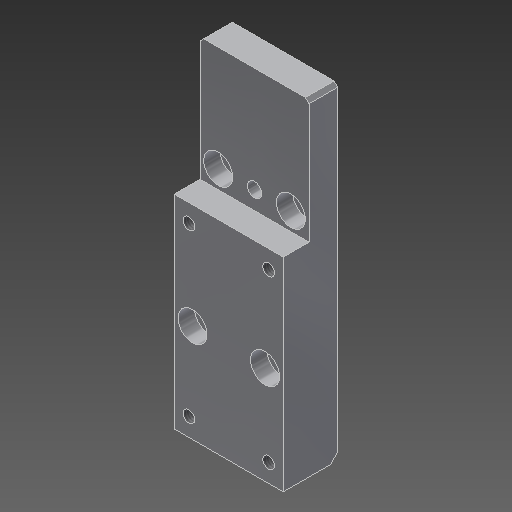
# Autodesk Inventor part: 04
Saved by Autodesk Inventor 2021.1 (Build 251245010, 245A)
## iProperties
Created: 2008-11-14
Part Number: 04
Document SubType Name: Modeling
Density: 2.71 g/cm^3
Material: A5052
Mass: 48.5632 g
Surface Area: 53.44 cm^2
Volume: 17.92 cm^3
Appearance: アルミニウム - フラット
個数: 1
尺度: 1:1
Title: プレート
Autodesk Inventor part; units mm, degrees
ref_plane "YZ Plane" through (0, 0, 0) normal (1, 0, 0) x (0, 1, 0)
ref_plane "XZ Plane" through (0, 0, 0) normal (0, 1, 0) x (-1, 0, 0)
ref_plane "XY Plane" through (0, 0, 0) normal (0, 0, 1) x (1, 0, 0)
sketch "スケッチ1" plane through (0, 0, 0) normal (0, 0, 1) x (1, 0, 0)
  line L0 (-15, -45) -> (15, -45)
  line L1 (15, -45) -> (15, 45)
  line L2 (15, 45) -> (-15, 45)
  line L3 (-15, 45) -> (-15, -45)
  point P0 (0, 0)
  point P1 (0, -45)
  point P2 (-15, 0)
  dimension "d0" = 30
  dimension "d1" = 90
  constraints: 8 end point, 2 midpoint, 2 parallel, 1 horizontal, 1 horizontal alignment, 1 perpendicular, 1 vertical alignment
  measures "d0" distance of L0.start L0.end
  measures "d1" distance of L2.end L0.start
extrude "押し出し1" add sketch "スケッチ1" along normal blind 15
sketch "スケッチ6" plane through (0, 0, 15) normal (0, 0, 1) x (1, 0, 0)
  line L0 (15, -45) -> (-15, -45) projected
  point P0 (0, 0)
  point P1 (-11, -40)
  dimension "d33" = 11
  dimension "d52" = 5
  measures "d33" horizontal distance of point (-11, -40) point (0, 0)
  measures "d52" distance from line of point (-11, -40) L0
hole "穴3" at (-11, -40, 15) direction (0, 0, -1) diameter 3.242 end through all thread size "M4x0.7" class "6H" standard "ANSI Metric M Profile"
pattern_linear "矩形状パターン2" count 2 spacing 22 along (1, 0, 0) count 2 spacing 46 along (0, 1, 0) of "穴3"
sketch "スケッチ9" plane through (0, 0, 15) normal (0, 0, 1) x (1, 0, 0)
  line L0 (15, -45) -> (-15, -45) projected
  point P0 (0, 0)
  point P1 (-10, -18)
  point P2 (10, -18)
  dimension "d53" = 27
  dimension "d54" = 10
  dimension "d62" = 10
  constraints: 1 horizontal alignment
  measures "d53" distance from line of point (-10, -18) L0
  measures "d54" horizontal distance of point (-10, -18) point (0, 0)
  measures "d62" horizontal distance of point (10, -18) point (0, 0)
hole "穴4" at (-10, -18, 15) at (10, -18, 15) direction (0, 0, -1) diameter 4.5 end through all counterbore diameter 8 counterbore depth 4.5
sketch "スケッチ10" plane through (0, 0, 15) normal (0, 0, 1) x (1, 0, 0)
  circle A0 centre (-11, 6) radius 1.621 projected
  line L0 (-15, -45) -> (-15, 45) projected
  line L1 (15, 45) -> (15, -45) projected
  line L2 (-15, 45) -> (15, 45) projected
  line L3 (-15, 11) -> (15, 11)
  point P0 (0, 0)
  dimension "d63" = 5
  constraints: 2 end point, 2 point on line, 1 horizontal
  measures "d63" distance from line of L3 A0.centre
extrude "押し出し5" cut sketch "スケッチ10" against normal blind 7.1 contours L0 L2 L1 L3
sketch "スケッチ11" plane through (0, 0, 7.9) normal (0, 0, 1) x (1, 0, 0)
  circle A0 centre (-10, -18) radius 4 projected
  circle A1 centre (10, -18) radius 4 projected
  point P0 (0, 0)
  point P1 (-10, 16)
  point P2 (10, 16)
  dimension "d66" = 34
  constraints: 2 vertical alignment, 1 horizontal alignment
  measures "d66" distance of point (-10, 16) A0.centre
hole "穴5" at (-10, 16, 7.9) at (10, 16, 7.9) direction (0, 0, -1) diameter 4.5 end through all counterbore diameter 8 counterbore depth 4.5
chamfer "面取り1" distance 1 angle 45 2 edges at (15, 45, 3.95) (-15, 45, 3.95)
sketch "スケッチ12" plane through (0, 0, 0) normal (0, 0, -1) x (-1, 0, 0)
  line L0 (15, -45) -> (-15, -45) projected
  circle A0 centre (-10, 16) radius 2.25 projected
  circle A1 centre (-10, -18) radius 2.25 projected
  point P0 (0, 0)
  point P1 (0, 16)
  point P2 (0, -18)
  point P3 (0, -45)
  constraints: 2 horizontal alignment, 2 vertical alignment, 1 midpoint
hole "穴6" at (0, 16, 0) at (0, -18, 0) direction (0, 0, 1) diameter 4 depth 8 tip angle 118
chamfer "面取り2" distance 2 angle 45 1 edges at (0, -45, 0)
equation "\"d62\" = d54"
